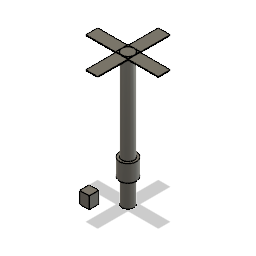
_camara top.273ecf29-dca3-4243-8d60-dc86f891365d (Autodesk Fusion 360 design; units mm, degrees)
Autodesk Fusion 360 part; units mm, degrees
note: some values were not read from the file. Chosen so that the rebuilt part matches the saved one: which bodies a step acts on.
sketch "Sketch1" plane through (0, 0, 0) normal (0, 1, 0) x (1, 0, 0)
  circle A0 centre (0, 0) radius 25
  circle A1 centre (0, 0) radius 35
  dimension "d1" = 50
  dimension "d2" = 70
  measures "d1" diameter of A0
  measures "d2" diameter of A1
extrude "Extrude1" add sketch "Sketch1" along normal blind 375 contours A0 makes body 1
extrude "Extrude2" add sketch "Sketch1" along normal blind 70 separate body contours A0 | A1 makes body 2
extrude "Extrude3" add sketch "Sketch1" along normal blind 100 separate body contours A0 makes body 3
sketch "Sketch2" plane through (0, 0, 0) normal (0, 1, 0) x (1, 0, 0)
  line L0 (20, 20) -> (-20, 20)
  line L1 (-20, 20) -> (-20, -20)
  line L2 (-20, -20) -> (20, -20)
  line L3 (20, -20) -> (20, 20)
  line L4 (20, 20) -> (-20, -20) construction
  line L5 (-20, 20) -> (20, -20) construction
  dimension "d9" = 40
  dimension "d10" = 40
  measures "d9" distance of L0.end L1.end
  measures "d10" distance of L1.end L2.end
extrude "Extrude6" add sketch "Sketch2" along normal blind 50 separate body makes body 4
copy_body "Body->Comp2" bodies 1 removing the originals makes body 5 in component "Component"
copy_body "Body->Comp3" bodies 3 removing the originals makes body 6 in component "Component'"
copy_body "Body->Comp4" bodies 2 removing the originals makes body 7 in component "Component''"
copy_body "Body->Comp5" bodies 4 removing the originals makes body 8 in component "Component'''"
sketch "Sketch3" plane through (0, 0, 0) normal (0, 1, 0) x (1, 0, 0)
  line L0 (25, 150) -> (-25, 150)
  line L1 (-25, 150) -> (-25, -150)
  line L2 (-25, -150) -> (25, -150)
  line L3 (25, -150) -> (25, 150)
  line L4 (25, 150) -> (-25, -150) construction
  line L5 (-25, 150) -> (25, -150) construction
  line L6 (150, 25) -> (-150, 25)
  line L7 (-150, 25) -> (-150, -25)
  line L8 (-150, -25) -> (150, -25)
  line L9 (150, -25) -> (150, 25)
  line L10 (150, 25) -> (-150, -25) construction
  line L11 (-150, 25) -> (150, -25) construction
  dimension "d17" = 300
  dimension "d18" = 50
  dimension "d19" = 300
  dimension "d20" = 50
  measures "d17" distance of L0.end L1.end
  measures "d18" distance of L1.end L2.end
  measures "d19" distance of L7.end L8.end
  measures "d20" distance of L6.end L7.end
extrude "Extrude7" add sketch "Sketch3" sketch "Sketch2" along normal blind 3 separate body contours L0 L1 L3 L6 | L3 L6 L8 L9 | L1 L6 L7 L8 | L1 L2 L3 L8 of sketch 2 makes body 9 at (8.3333, 0, -66.6667) makes body 9 at (66.6667, 0, -8.3333) makes body 9 at (-108.3333, 0, -8.3333) makes body 9 at (-8.3333, 0, 108.3333) makes body 10 at (-6.6667, 0, -6.6667)
extrude "Extrude8" add sketch "Sketch3" along normal blind 5 contours L1 L3 L6 L8 bodies 9
copy_body "Body->Comp6" bodies 9 removing the originals makes body 11 in component "Component''''"
component "Component" placed x (1, 0, 0) y (0, 1, 0) z (0, 0, 1) at (0, 170, 0)
component "Component'" placed x (1, 0, 0) y (0, 1, 0) z (0, 0, 1) at (0, 0, 0)
component "Component''" placed x (1, 0, 0) y (0, 1, 0) z (0, 0, 1) at (0, 100, 0)
component "Component'''" placed x (1, 0, 0) y (0, 1, 0) z (0, 0, 1) at (-80, 0, 80)
component "Component''''" placed x (1, 0, 0) y (0, 1, 0) z (0, 0, 1) at (0, 0, 0)
hidden bodies 10
